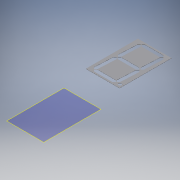
# Autodesk Inventor part: Cover_V2
Saved by Autodesk Inventor 2016 SP2 (Build 200236200, 236)
## iProperties
Created: 2018-06-10
Part Number: Cover_V2
Material: Generisch
Document SubType Name: Modeling
Designer: Nils
Density: 1 g/cm^3
Appearance: Vorgabe
Author: Nils
Autodesk Inventor part; units mm, degrees
ref_plane "YZ Plane" through (0, 0, 0) normal (1, 0, 0) x (0, 1, 0)
ref_plane "XZ Plane" through (0, 0, 0) normal (0, 1, 0) x (-1, 0, 0)
ref_plane "XY Plane" through (0, 0, 0) normal (0, 0, 1) x (1, 0, 0)
sketch "Skizze1" plane through (0, 0, 0) normal (0, 0, 1) x (1, 0, 0)
  line L0 (-29.0874, 344.6415) -> (-29.0874, 191.4405) projected
  line L1 (-29.0874, 191.4405) -> (69.9128, 191.4405) projected
  line L2 (-21.0874, 207.6072) -> (-18.2612, 261.5332) projected
  line L3 (-16.0874, 202.6072) -> (-21.0874, 207.6072) projected
  line L4 (-11.0874, 207.6072) -> (-16.0874, 202.6072) projected
  line L5 (-18.2612, 261.5332) -> (-13.2612, 266.5332) projected
  line L6 (-13.2612, 266.5332) -> (-8.2612, 261.5332) projected
  line L7 (44.0794, 196.4405) -> (-9.9206, 196.4405) projected
  line L8 (-9.9206, 196.4405) -> (-14.9206, 201.4405) projected
  line L9 (-14.9206, 201.4405) -> (-9.9206, 206.4405) projected
  line L10 (49.0794, 201.4405) -> (44.0794, 196.4405) projected
  line L11 (44.0794, 206.4405) -> (49.0794, 201.4405) projected
  line L12 (-9.9206, 206.4405) -> (44.0794, 206.4405)
  line L13 (-11.0874, 207.6072) -> (-8.2612, 261.5332)
  line L14 (-17.5791, 274.5488) -> (-14.753, 328.4748) projected
  line L15 (-12.5791, 269.5488) -> (-17.5791, 274.5488) projected
  line L16 (-7.5791, 274.5488) -> (-12.5791, 269.5488) projected
  line L17 (-14.753, 328.4748) -> (-9.753, 333.4748) projected
  line L18 (-9.753, 333.4748) -> (-4.753, 328.4748) projected
  line L19 (-3.5862, 329.6415) -> (-8.5862, 334.6415) projected
  line L20 (-8.5862, 334.6415) -> (-3.5862, 339.6415) projected
  line L21 (-3.5862, 339.6415) -> (50.4138, 339.6415) projected
  line L22 (50.4138, 339.6415) -> (55.4138, 334.6415) projected
  line L23 (55.4138, 334.6415) -> (50.4138, 329.6415) projected
  line L24 (51.5805, 328.4748) -> (56.5805, 333.4748) projected
  line L25 (56.5805, 333.4748) -> (61.5805, 328.4748) projected
  line L26 (61.5805, 328.4748) -> (58.7544, 274.5488) projected
  line L27 (58.7544, 274.5488) -> (53.7544, 269.5488) projected
  line L28 (53.7544, 269.5488) -> (48.7544, 274.5488) projected
  line L29 (-7.0945, 262.6999) -> (-12.0945, 267.6999) projected
  line L30 (-12.0945, 267.6999) -> (-7.0945, 272.6999) projected
  line L31 (-7.0945, 272.6999) -> (46.9055, 272.6999) projected
  line L32 (46.9055, 272.6999) -> (51.9055, 267.6999) projected
  line L33 (51.9055, 267.6999) -> (46.9055, 262.6999) projected
  line L34 (48.0722, 261.5332) -> (53.0722, 266.5332) projected
  line L35 (53.0722, 266.5332) -> (58.0722, 261.5332) projected
  line L36 (58.0722, 261.5332) -> (55.2461, 207.6072) projected
  line L37 (55.2461, 207.6072) -> (50.2461, 202.6072) projected
  line L38 (50.2461, 202.6072) -> (45.2461, 207.6072) projected
  line L39 (64.7975, 194.589) -> (50.5282, 194.589) construction
  line L40 (56.4128, 206.4405) -> (66.9128, 206.4405) construction
  line L41 (66.9128, 206.4405) -> (66.9128, 196.4405) construction
  line L42 (48.4128, 194.589) -> (48.4128, 196.4405) construction
  circle A0 centre (60.9128, 201.9405) radius 4.5
  line L43 (45.2461, 207.6072) -> (48.0722, 261.5332)
  line L44 (46.9055, 262.6999) -> (-7.0945, 262.6999)
  line L45 (-7.5791, 274.5488) -> (-4.753, 328.4748)
  line L46 (-3.5862, 329.6415) -> (50.4138, 329.6415)
  line L47 (51.5805, 328.4748) -> (48.7544, 274.5488)
  line L48 (69.9128, 344.6415) -> (-29.0874, 344.6415) projected
  line L49 (69.9128, 191.4405) -> (69.9128, 344.6415) projected
  point P0 (0, 0)
  dimension "d2" = 9
  dimension "d3" = 4.5
  dimension "d4" = 4.5
  constraints: 14 end point, 4 point on line, 2 horizontal, 2 parallel, 1 centre point
  measures "d2" diameter of A0
  measures "d3" distance from line of L40 A0.centre
  measures "d4" horizontal distance of A0.centre L40.start
extrude "Extrusion2" add sketch "Skizze1" along normal blind 0.6
sketch "Skizze2" plane through (0, 0, 0) normal (0, 0, -1) x (-1, 0, 0)
  circle A0 centre (24.0874, 196.4405) radius 2.5 construction
  circle A1 centre (-64.9128, 267.6999) radius 2.5 construction
  circle A2 centre (24.0874, 267.6999) radius 2.5 construction
  circle A3 centre (24.0874, 339.6415) radius 2.5 construction
  circle A4 centre (-64.9128, 339.6415) radius 2.5 construction
  circle A5 centre (-64.9128, 267.6999) radius 2.4
  circle A6 centre (-64.9128, 339.6415) radius 2.4
  circle A7 centre (24.0874, 339.6415) radius 2.4
  circle A8 centre (24.0874, 267.6999) radius 2.4
  circle A9 centre (24.0874, 196.4405) radius 2.4
  point P0 (0, 0)
  dimension "d7" = 4.8
  dimension "d8" = 4.8
  dimension "d9" = 4.8
  dimension "d10" = 4.8
  dimension "d11" = 4.8
  constraints: 5 centre point, 5 coincident
  measures "d7" diameter of A5
  measures "d8" diameter of A6
  measures "d9" diameter of A7
  measures "d10" diameter of A8
  measures "d11" diameter of A9
extrude "Extrusion3" add sketch "Skizze2" along normal blind 2.6
ref_plane "Arbeitsebene1" through (20.4127, 47.5501, -21.1283) normal (0, 0, -1) x (-1, 0, 0)
equation "\"d4\" = d3"
equation "\"d8\" = d7"
equation "\"d9\" = d7"
equation "\"d10\" = d7"
equation "\"d11\" = d7"
